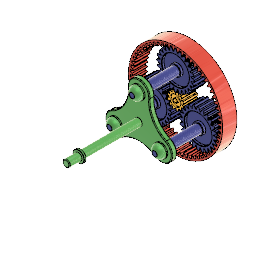
planetry gear v0 (Autodesk Fusion 360 design; units mm, degrees)
Autodesk Fusion 360 part; units mm, degrees
(part 1 of 2)
sketch "Sketch1" plane through (0, 0, 0) normal (0, 1, 0) x (1, 0, 0)
  arc A0 (-7.4766, -17.4075) -> (-18.8136, 2.2289) centre (-27.4141, -15.8275) ccw
  arc A1 (18.8136, 2.2289) -> (7.4766, -17.4075) centre (27.4141, -15.8275) ccw
  arc A2 (-11.3371, 15.1786) -> (11.3371, 15.1786) centre (0, 31.655) ccw
  arc A3 (18.8136, 2.2289) -> (11.3371, 15.1786) centre (15.5885, 9) ccw
  arc A4 (-11.3371, 15.1786) -> (-18.8136, 2.2289) centre (-15.5885, 9) ccw
  arc A5 (-7.4766, -17.4075) -> (7.4766, -17.4075) centre (0, -18) ccw
  circle A6 centre (0, -18) radius 4.5
  circle A7 centre (15.5885, 9) radius 4.5
  circle A8 centre (-15.5885, 9) radius 4.5
  circle A9 centre (0, 0) radius 2.5
  dimension "d1" = 18
  dimension "d2" = 15
  dimension "d5" = 40
  dimension "d6" = 40
  dimension "d7" = 9
  dimension "d9" = 360
  dimension "d10" = 5
  constraint tangent A1 A5
  constraint tangent A1 A3
  constraint tangent A2 A3
  constraint tangent A2 A4
  constraint concentric A5 A6
  constraint coincident A9.centre origin
  measures "d1" distance of A9.centre A5.centre
  measures "d2" diameter of A5
  measures "d5" diameter of A1
  measures "d6" diameter of A2
  measures "d7" diameter of A6
  measures "d10" diameter of A9
extrude "Extrude1" add sketch "Sketch1" along normal blind 3.5 makes body 1
extrude "Extrude2" add sketch "Sketch1" against normal blind 50 separate body contours A9 makes body 2
ref_plane "WorkPlane1" through (0, -40, 0) normal (0, 1, 0) x (0, 0, 1)
sketch "Sketch2" plane through (0, -40, 0) normal (0, 1, 0) x (1, 0, 0)
  circle A0 centre (0, 0) radius 4
  dimension "d16" = 8
  constraint coincident A0.centre origin
  measures "d16" diameter of A0
extrude "Extrude3" add sketch "Sketch2" against normal blind 1.5 bodies 2
fillet "Fillet1" radius 0.5 12 edges at (22.0836, 3.5, -12.75) (0, 3.5, -11.655) (-22.0836, 3.5, -12.75) (-10.0935, 3.5, 5.8275) (0, 3.5, 25.5) (10.0935, 3.5, 5.8275) (0, 0, 25.5) (-10.0935, 0, 5.8275) (-22.0836, 0, -12.75) (0, 0, -11.655) (22.0836, 0, -12.75) (10.0935, 0, 5.8275) on bodies 1
fillet "Fillet2" radius 0.2 2 edges at (-3.7293, -40, 1.4465) (-3.7293, -41.5, -1.4465) on bodies 2
chamfer "Chamfer1" distance 0.5 angle 45 1 edges at (-2.3308, -50, -0.904) measured on face at (-0.8863, -50, -0.2321) on bodies 2
ref_plane "WorkPlane2" through (0, 35.45, 0) normal (0, 1, 0) x (0, 0, 1)
sketch "Sketch3" plane through (0, 35.45, 0) normal (0, 1, 0) x (1, 0, 0)
  line L0 (0.5196, -30.9896) -> (0.9976, -29.763)
  arc A0 (0.9976, -29.763) -> (1.2198, -28.6806) centre (-2.0612, -28.571) ccw
  line L1 (0, -31.1) -> (0, -31.7)
  line L2 (-0.5196, -30.9896) -> (-0.9976, -29.763)
  arc A1 (-1.2198, -28.6806) -> (-0.9976, -29.763) centre (2.0612, -28.571) ccw
  arc A2 (-0.5196, -30.9896) -> (0.5196, -30.9896) centre (0, -18) ccw
  arc A3 (4.0081, -29.104) -> (3.9426, -28.0009) centre (0.745, -28.7442) ccw
  line L3 (3.8638, -30.4125) -> (4.0081, -29.104)
  arc A4 (2.8601, -30.6815) -> (3.8638, -30.4125) centre (0, -18) ccw
  line L4 (2.8601, -30.6815) -> (2.0809, -29.6204)
  arc A5 (1.5861, -28.6324) -> (2.0809, -29.6204) centre (4.7269, -27.6773) ccw
  arc A6 (6.7454, -27.6882) -> (6.3967, -26.6397) centre (3.5005, -28.1853) ccw
  line L5 (6.9448, -28.9895) -> (6.7454, -27.6882)
  arc A7 (6.0448, -29.5091) -> (6.9448, -28.9895) centre (0, -18) ccw
  line L6 (6.0448, -29.5091) -> (5.0175, -28.6858)
  arc A8 (4.2839, -27.8596) -> (5.0175, -28.6858) centre (7.0705, -26.1241) ccw
  arc A9 (9.0231, -25.6123) -> (8.4149, -24.6897) centre (6.0173, -26.9323) ccw
  line L7 (9.5524, -26.8176) -> (9.0231, -25.6123)
  arc A10 (8.8176, -27.5524) -> (9.5524, -26.8176) centre (0, -18) ccw
  line L8 (8.8176, -27.5524) -> (7.6123, -27.0231)
  arc A11 (6.6897, -26.4149) -> (7.6123, -27.0231) centre (8.9323, -24.0173) ccw
  arc A12 (10.6858, -23.0175) -> (9.8596, -22.2839) centre (8.1241, -25.0705) ccw
  line L9 (11.5091, -24.0448) -> (10.6858, -23.0175)
  arc A13 (10.9895, -24.9448) -> (11.5091, -24.0448) centre (0, -18) ccw
  line L10 (10.9895, -24.9448) -> (9.6882, -24.7454)
  arc A14 (8.6397, -24.3967) -> (9.6882, -24.7454) centre (10.1853, -21.5005) ccw
  arc A15 (11.6204, -20.0809) -> (10.6324, -19.5861) centre (9.6773, -22.7269) ccw
  line L11 (12.6815, -20.8601) -> (11.6204, -20.0809)
  arc A16 (12.4125, -21.8638) -> (12.6815, -20.8601) centre (0, -18) ccw
  line L12 (12.4125, -21.8638) -> (11.104, -22.0081)
  arc A17 (10.0009, -21.9426) -> (11.104, -22.0081) centre (10.7442, -18.745) ccw
  arc A18 (11.763, -17.0024) -> (10.6806, -16.7802) centre (10.571, -20.0612) ccw
  line L13 (12.9896, -17.4804) -> (11.763, -17.0024)
  arc A19 (12.9896, -18.5196) -> (12.9896, -17.4804) centre (0, -18) ccw
  line L14 (12.9896, -18.5196) -> (11.763, -18.9976)
  arc A20 (10.6806, -19.2198) -> (11.763, -18.9976) centre (10.571, -15.9388) ccw
  arc A21 (11.104, -13.9919) -> (10.0009, -14.0574) centre (10.7442, -17.255) ccw
  line L15 (12.4125, -14.1362) -> (11.104, -13.9919)
  arc A22 (12.6815, -15.1399) -> (12.4125, -14.1362) centre (0, -18) ccw
  line L16 (12.6815, -15.1399) -> (11.6204, -15.9191)
  arc A23 (10.6324, -16.4139) -> (11.6204, -15.9191) centre (9.6773, -13.2731) ccw
  arc A24 (9.6882, -11.2546) -> (8.6397, -11.6033) centre (10.1853, -14.4995) ccw
  line L17 (10.9895, -11.0552) -> (9.6882, -11.2546)
  arc A25 (11.5091, -11.9552) -> (10.9895, -11.0552) centre (0, -18) ccw
  line L18 (11.5091, -11.9552) -> (10.6858, -12.9825)
  arc A26 (9.8596, -13.7161) -> (10.6858, -12.9825) centre (8.1241, -10.9295) ccw
  arc A27 (7.6123, -8.9769) -> (6.6897, -9.5851) centre (8.9323, -11.9827) ccw
  line L19 (8.8176, -8.4476) -> (7.6123, -8.9769)
  arc A28 (9.5524, -9.1824) -> (8.8176, -8.4476) centre (0, -18) ccw
  line L20 (9.5524, -9.1824) -> (9.0231, -10.3877)
  arc A29 (8.4149, -11.3103) -> (9.0231, -10.3877) centre (6.0173, -9.0677) ccw
  arc A30 (5.0175, -7.3142) -> (4.2839, -8.1404) centre (7.0705, -9.8759) ccw
  line L21 (6.0448, -6.4909) -> (5.0175, -7.3142)
  arc A31 (6.9448, -7.0105) -> (6.0448, -6.4909) centre (0, -18) ccw
  line L22 (6.9448, -7.0105) -> (6.7454, -8.3118)
  arc A32 (6.3967, -9.3603) -> (6.7454, -8.3118) centre (3.5005, -7.8147) ccw
  arc A33 (2.0809, -6.3796) -> (1.5861, -7.3676) centre (4.7269, -8.3227) ccw
  line L23 (2.8601, -5.3185) -> (2.0809, -6.3796)
  arc A34 (3.8638, -5.5875) -> (2.8601, -5.3185) centre (0, -18) ccw
  line L24 (3.8638, -5.5875) -> (4.0081, -6.896)
  arc A35 (3.9426, -7.9991) -> (4.0081, -6.896) centre (0.745, -7.2558) ccw
  arc A36 (-0.9976, -6.237) -> (-1.2198, -7.3194) centre (2.0612, -7.429) ccw
  line L25 (-0.5196, -5.0104) -> (-0.9976, -6.237)
  arc A37 (0.5196, -5.0104) -> (-0.5196, -5.0104) centre (0, -18) ccw
  line L26 (0.5196, -5.0104) -> (0.9976, -6.237)
  arc A38 (1.2198, -7.3194) -> (0.9976, -6.237) centre (-2.0612, -7.429) ccw
  arc A39 (-4.0081, -6.896) -> (-3.9426, -7.9991) centre (-0.745, -7.2558) ccw
  line L27 (-3.8638, -5.5875) -> (-4.0081, -6.896)
  arc A40 (-2.8601, -5.3185) -> (-3.8638, -5.5875) centre (0, -18) ccw
  line L28 (-2.8601, -5.3185) -> (-2.0809, -6.3796)
  arc A41 (-1.5861, -7.3676) -> (-2.0809, -6.3796) centre (-4.7269, -8.3227) ccw
  arc A42 (-6.7454, -8.3118) -> (-6.3967, -9.3603) centre (-3.5005, -7.8147) ccw
  line L29 (-6.9448, -7.0105) -> (-6.7454, -8.3118)
  arc A43 (-6.0448, -6.4909) -> (-6.9448, -7.0105) centre (0, -18) ccw
  line L30 (-6.0448, -6.4909) -> (-5.0175, -7.3142)
  arc A44 (-4.2839, -8.1404) -> (-5.0175, -7.3142) centre (-7.0705, -9.8759) ccw
  arc A45 (-9.0231, -10.3877) -> (-8.4149, -11.3103) centre (-6.0173, -9.0677) ccw
  line L31 (-9.5524, -9.1824) -> (-9.0231, -10.3877)
  arc A46 (-8.8176, -8.4476) -> (-9.5524, -9.1824) centre (0, -18) ccw
  line L32 (-8.8176, -8.4476) -> (-7.6123, -8.9769)
  arc A47 (-6.6897, -9.5851) -> (-7.6123, -8.9769) centre (-8.9323, -11.9827) ccw
  arc A48 (-10.6858, -12.9825) -> (-9.8596, -13.7161) centre (-8.1241, -10.9295) ccw
  line L33 (-11.5091, -11.9552) -> (-10.6858, -12.9825)
  arc A49 (-10.9895, -11.0552) -> (-11.5091, -11.9552) centre (0, -18) ccw
  line L34 (-10.9895, -11.0552) -> (-9.6882, -11.2546)
  arc A50 (-8.6397, -11.6033) -> (-9.6882, -11.2546) centre (-10.1853, -14.4995) ccw
  arc A51 (-11.6204, -15.9191) -> (-10.6324, -16.4139) centre (-9.6773, -13.2731) ccw
  line L35 (-12.6815, -15.1399) -> (-11.6204, -15.9191)
  arc A52 (-12.4125, -14.1362) -> (-12.6815, -15.1399) centre (0, -18) ccw
  line L36 (-12.4125, -14.1362) -> (-11.104, -13.9919)
  arc A53 (-10.0009, -14.0574) -> (-11.104, -13.9919) centre (-10.7442, -17.255) ccw
  arc A54 (-11.763, -18.9976) -> (-10.6806, -19.2198) centre (-10.571, -15.9388) ccw
  line L37 (-12.9896, -18.5196) -> (-11.763, -18.9976)
  arc A55 (-12.9896, -17.4804) -> (-12.9896, -18.5196) centre (0, -18) ccw
  line L38 (-12.9896, -17.4804) -> (-11.763, -17.0024)
  arc A56 (-10.6806, -16.7802) -> (-11.763, -17.0024) centre (-10.571, -20.0612) ccw
  arc A57 (-11.104, -22.0081) -> (-10.0009, -21.9426) centre (-10.7442, -18.745) ccw
  line L39 (-12.4125, -21.8638) -> (-11.104, -22.0081)
  arc A58 (-12.6815, -20.8601) -> (-12.4125, -21.8638) centre (0, -18) ccw
  line L40 (-12.6815, -20.8601) -> (-11.6204, -20.0809)
  arc A59 (-10.6324, -19.5861) -> (-11.6204, -20.0809) centre (-9.6773, -22.7269) ccw
  arc A60 (-9.6882, -24.7454) -> (-8.6397, -24.3967) centre (-10.1853, -21.5005) ccw
  line L41 (-10.9895, -24.9448) -> (-9.6882, -24.7454)
  arc A61 (-11.5091, -24.0448) -> (-10.9895, -24.9448) centre (0, -18) ccw
  line L42 (-11.5091, -24.0448) -> (-10.6858, -23.0175)
  arc A62 (-9.8596, -22.2839) -> (-10.6858, -23.0175) centre (-8.1241, -25.0705) ccw
  arc A63 (-7.6123, -27.0231) -> (-6.6897, -26.4149) centre (-8.9323, -24.0173) ccw
  line L43 (-8.8176, -27.5524) -> (-7.6123, -27.0231)
  arc A64 (-9.5524, -26.8176) -> (-8.8176, -27.5524) centre (0, -18) ccw
  line L44 (-9.5524, -26.8176) -> (-9.0231, -25.6123)
  arc A65 (-8.4149, -24.6897) -> (-9.0231, -25.6123) centre (-6.0173, -26.9323) ccw
  arc A66 (-5.0175, -28.6858) -> (-4.2839, -27.8596) centre (-7.0705, -26.1241) ccw
  line L45 (-6.0448, -29.5091) -> (-5.0175, -28.6858)
  arc A67 (-6.9448, -28.9895) -> (-6.0448, -29.5091) centre (0, -18) ccw
  line L46 (-6.9448, -28.9895) -> (-6.7454, -27.6882)
  arc A68 (-6.3967, -26.6397) -> (-6.7454, -27.6882) centre (-3.5005, -28.1853) ccw
  arc A69 (-2.0809, -29.6204) -> (-1.5861, -28.6324) centre (-4.7269, -27.6773) ccw
  line L47 (-2.8601, -30.6815) -> (-2.0809, -29.6204)
  arc A70 (-3.8638, -30.4125) -> (-2.8601, -30.6815) centre (0, -18) ccw
  line L48 (-3.8638, -30.4125) -> (-4.0081, -29.104)
  arc A71 (-3.9426, -28.0009) -> (-4.0081, -29.104) centre (-0.745, -28.7442) ccw
  arc A72 (-1.5861, -28.6324) -> (-1.2198, -28.6806) centre (0, -18) ccw
  arc A73 (1.2198, -28.6806) -> (1.5861, -28.6324) centre (0, -18) ccw
  arc A74 (-4.2839, -27.8596) -> (-3.9426, -28.0009) centre (0, -18) ccw
  arc A75 (-6.6897, -26.4149) -> (-6.3967, -26.6397) centre (0, -18) ccw
  arc A76 (3.9426, -28.0009) -> (4.2839, -27.8596) centre (0, -18) ccw
  arc A77 (6.3967, -26.6397) -> (6.6897, -26.4149) centre (0, -18) ccw
  arc A78 (8.4149, -24.6897) -> (8.6397, -24.3967) centre (0, -18) ccw
  arc A79 (9.8596, -22.2839) -> (10.0009, -21.9426) centre (0, -18) ccw
  arc A80 (10.6324, -19.5861) -> (10.6806, -19.2198) centre (0, -18) ccw
  arc A81 (10.6806, -16.7802) -> (10.6324, -16.4139) centre (0, -18) ccw
  arc A82 (10.0009, -14.0574) -> (9.8596, -13.7161) centre (0, -18) ccw
  arc A83 (8.6397, -11.6033) -> (8.4149, -11.3103) centre (0, -18) ccw
  arc A84 (6.6897, -9.5851) -> (6.3967, -9.3603) centre (0, -18) ccw
  arc A85 (4.2839, -8.1404) -> (3.9426, -7.9991) centre (0, -18) ccw
  arc A86 (1.5861, -7.3676) -> (1.2198, -7.3194) centre (0, -18) ccw
  arc A87 (-1.2198, -7.3194) -> (-1.5861, -7.3676) centre (0, -18) ccw
  arc A88 (-3.9426, -7.9991) -> (-4.2839, -8.1404) centre (0, -18) ccw
  arc A89 (-6.3967, -9.3603) -> (-6.6897, -9.5851) centre (0, -18) ccw
  arc A90 (-8.4149, -11.3103) -> (-8.6397, -11.6033) centre (0, -18) ccw
  arc A91 (-9.8596, -13.7161) -> (-10.0009, -14.0574) centre (0, -18) ccw
  arc A92 (-10.6324, -16.4139) -> (-10.6806, -16.7802) centre (0, -18) ccw
  arc A93 (-10.6806, -19.2198) -> (-10.6324, -19.5861) centre (0, -18) ccw
  arc A94 (-10.0009, -21.9426) -> (-9.8596, -22.2839) centre (0, -18) ccw
  arc A95 (-8.6397, -24.3967) -> (-8.4149, -24.6897) centre (0, -18) ccw
  circle A96 centre (0, -18) radius 3
  dimension "d26" = 26
  dimension "d28" = 21.5
  dimension "d32" = 360
  dimension "d33" = 6
  constraint concentric A2 A72
  constraint coincident A0.end A72
  constraint tangent L0 A0
  constraint vertical L1
  constraint symmetric L0.start L1 L2.start
  constraint symmetric L0.end L1 L2.end
  constraint symmetric A0.end L1 A1.start
  constraint symmetric A0 L1 A1
  constraint concentric A72 A73
  constraint concentric A73 A76
  constraint concentric A74 A76
  constraint concentric A75 A76
  constraint concentric A76 A77
  constraint concentric A77 A78
  constraint concentric A78 A79
  constraint concentric A79 A80
  constraint concentric A80 A81
  constraint concentric A81 A82
  constraint concentric A82 A83
  constraint concentric A83 A84
  constraint concentric A84 A85
  constraint concentric A85 A86
  constraint concentric A86 A87
  constraint concentric A87 A88
  constraint concentric A88 A89
  constraint concentric A89 A90
  constraint concentric A90 A91
  constraint concentric A91 A92
  constraint concentric A92 A93
  constraint concentric A93 A94
  constraint concentric A94 A95
  constraint concentric A22 A96
  measures "d26" diameter of A2
  measures "d28" diameter of A72
  measures "d33" diameter of A96
extrude "Extrude4" add sketch "Sketch3" against normal blind 10 separate body makes body 3
sketch "Sketch4" plane through (0, 25.45, 0) normal (0, -1, 0) x (1, 0, 0)
  circle A0 centre (0, 18) radius 3
  arc A1 (-10.9895, 24.9448) -> (-11.5091, 24.0448) centre (0, 18) ccw
  line L0 (-11.5091, 24.0448) -> (-10.6858, 23.0175)
  arc A2 (-10.6858, 23.0175) -> (-9.8596, 22.2839) centre (-8.1241, 25.0705) ccw
  arc A3 (-9.8596, 22.2839) -> (-10.0009, 21.9426) centre (0, 18) ccw
  arc A4 (-10.0009, 21.9426) -> (-11.104, 22.0081) centre (-10.7442, 18.745) ccw
  line L1 (-11.104, 22.0081) -> (-12.4125, 21.8638)
  arc A5 (-12.4125, 21.8638) -> (-12.6815, 20.8601) centre (0, 18) ccw
  line L2 (-12.6815, 20.8601) -> (-11.6204, 20.0809)
  arc A6 (-11.6204, 20.0809) -> (-10.6324, 19.5861) centre (-9.6773, 22.7269) ccw
  arc A7 (-10.6324, 19.5861) -> (-10.6806, 19.2198) centre (0, 18) ccw
  arc A8 (-10.6806, 19.2198) -> (-11.763, 18.9976) centre (-10.571, 15.9388) ccw
  line L3 (-11.763, 18.9976) -> (-12.9896, 18.5196)
  arc A9 (-12.9896, 18.5196) -> (-12.9896, 17.4804) centre (0, 18) ccw
  line L4 (-12.9896, 17.4804) -> (-11.763, 17.0024)
  arc A10 (-11.763, 17.0024) -> (-10.6806, 16.7802) centre (-10.571, 20.0612) ccw
  arc A11 (-10.6806, 16.7802) -> (-10.6324, 16.4139) centre (0, 18) ccw
  arc A12 (-10.6324, 16.4139) -> (-11.6204, 15.9191) centre (-9.6773, 13.2731) ccw
  line L5 (-11.6204, 15.9191) -> (-12.6815, 15.1399)
  arc A13 (-12.6815, 15.1399) -> (-12.4125, 14.1362) centre (0, 18) ccw
  line L6 (-12.4125, 14.1362) -> (-11.104, 13.9919)
  arc A14 (-11.104, 13.9919) -> (-10.0009, 14.0574) centre (-10.7442, 17.255) ccw
  arc A15 (-10.0009, 14.0574) -> (-9.8596, 13.7161) centre (0, 18) ccw
  arc A16 (-9.8596, 13.7161) -> (-10.6858, 12.9825) centre (-8.1241, 10.9295) ccw
  line L7 (-10.6858, 12.9825) -> (-11.5091, 11.9552)
  arc A17 (-11.5091, 11.9552) -> (-10.9895, 11.0552) centre (0, 18) ccw
  line L8 (-10.9895, 11.0552) -> (-9.6882, 11.2546)
  arc A18 (-9.6882, 11.2546) -> (-8.6397, 11.6033) centre (-10.1853, 14.4995) ccw
  arc A19 (-8.6397, 11.6033) -> (-8.4149, 11.3103) centre (0, 18) ccw
  arc A20 (-8.4149, 11.3103) -> (-9.0231, 10.3877) centre (-6.0173, 9.0677) ccw
  line L9 (-9.0231, 10.3877) -> (-9.5524, 9.1824)
  arc A21 (-9.5524, 9.1824) -> (-8.8176, 8.4476) centre (0, 18) ccw
  line L10 (-8.8176, 8.4476) -> (-7.6123, 8.9769)
  arc A22 (-7.6123, 8.9769) -> (-6.6897, 9.5851) centre (-8.9323, 11.9827) ccw
  arc A23 (-6.6897, 9.5851) -> (-6.3967, 9.3603) centre (0, 18) ccw
  arc A24 (-6.3967, 9.3603) -> (-6.7454, 8.3118) centre (-3.5005, 7.8147) ccw
  line L11 (-6.7454, 8.3118) -> (-6.9448, 7.0105)
  arc A25 (-6.9448, 7.0105) -> (-6.0448, 6.4909) centre (0, 18) ccw
  line L12 (-6.0448, 6.4909) -> (-5.0175, 7.3142)
  arc A26 (-5.0175, 7.3142) -> (-4.2839, 8.1404) centre (-7.0705, 9.8759) ccw
  arc A27 (-4.2839, 8.1404) -> (-3.9426, 7.9991) centre (0, 18) ccw
  arc A28 (-3.9426, 7.9991) -> (-4.0081, 6.896) centre (-0.745, 7.2558) ccw
  line L13 (-4.0081, 6.896) -> (-3.8638, 5.5875)
  arc A29 (-3.8638, 5.5875) -> (-2.8601, 5.3185) centre (0, 18) ccw
  line L14 (-2.8601, 5.3185) -> (-2.0809, 6.3796)
  arc A30 (-2.0809, 6.3796) -> (-1.5861, 7.3676) centre (-4.7269, 8.3227) ccw
  arc A31 (-1.5861, 7.3676) -> (-1.2198, 7.3194) centre (0, 18) ccw
  arc A32 (-1.2198, 7.3194) -> (-0.9976, 6.237) centre (2.0612, 7.429) ccw
  line L15 (-0.9976, 6.237) -> (-0.5196, 5.0104)
  arc A33 (-0.5196, 5.0104) -> (0.5196, 5.0104) centre (0, 18) ccw
  line L16 (0.5196, 5.0104) -> (0.9976, 6.237)
  arc A34 (0.9976, 6.237) -> (1.2198, 7.3194) centre (-2.0612, 7.429) ccw
  arc A35 (1.2198, 7.3194) -> (1.5861, 7.3676) centre (0, 18) ccw
  arc A36 (1.5861, 7.3676) -> (2.0809, 6.3796) centre (4.7269, 8.3227) ccw
  line L17 (2.0809, 6.3796) -> (2.8601, 5.3185)
  arc A37 (2.8601, 5.3185) -> (3.8638, 5.5875) centre (0, 18) ccw
  line L18 (3.8638, 5.5875) -> (4.0081, 6.896)
  arc A38 (4.0081, 6.896) -> (3.9426, 7.9991) centre (0.745, 7.2558) ccw
  arc A39 (3.9426, 7.9991) -> (4.2839, 8.1404) centre (0, 18) ccw
  arc A40 (4.2839, 8.1404) -> (5.0175, 7.3142) centre (7.0705, 9.8759) ccw
  line L19 (5.0175, 7.3142) -> (6.0448, 6.4909)
  arc A41 (6.0448, 6.4909) -> (6.9448, 7.0105) centre (0, 18) ccw
  line L20 (6.9448, 7.0105) -> (6.7454, 8.3118)
  arc A42 (6.7454, 8.3118) -> (6.3967, 9.3603) centre (3.5005, 7.8147) ccw
  arc A43 (6.3967, 9.3603) -> (6.6897, 9.5851) centre (0, 18) ccw
  arc A44 (6.6897, 9.5851) -> (7.6123, 8.9769) centre (8.9323, 11.9827) ccw
  line L21 (7.6123, 8.9769) -> (8.8176, 8.4476)
  arc A45 (8.8176, 8.4476) -> (9.5524, 9.1824) centre (0, 18) ccw
  line L22 (9.5524, 9.1824) -> (9.0231, 10.3877)
  arc A46 (9.0231, 10.3877) -> (8.4149, 11.3103) centre (6.0173, 9.0677) ccw
  arc A47 (8.4149, 11.3103) -> (8.6397, 11.6033) centre (0, 18) ccw
  arc A48 (8.6397, 11.6033) -> (9.6882, 11.2546) centre (10.1853, 14.4995) ccw
  line L23 (9.6882, 11.2546) -> (10.9895, 11.0552)
  arc A49 (10.9895, 11.0552) -> (11.5091, 11.9552) centre (0, 18) ccw
  line L24 (11.5091, 11.9552) -> (10.6858, 12.9825)
  arc A50 (10.6858, 12.9825) -> (9.8596, 13.7161) centre (8.1241, 10.9295) ccw
  arc A51 (9.8596, 13.7161) -> (10.0009, 14.0574) centre (0, 18) ccw
  arc A52 (10.0009, 14.0574) -> (11.104, 13.9919) centre (10.7442, 17.255) ccw
  line L25 (11.104, 13.9919) -> (12.4125, 14.1362)
  arc A53 (12.4125, 14.1362) -> (12.6815, 15.1399) centre (0, 18) ccw
  line L26 (12.6815, 15.1399) -> (11.6204, 15.9191)
  arc A54 (11.6204, 15.9191) -> (10.6324, 16.4139) centre (9.6773, 13.2731) ccw
  arc A55 (10.6324, 16.4139) -> (10.6806, 16.7802) centre (0, 18) ccw
  arc A56 (10.6806, 16.7802) -> (11.763, 17.0024) centre (10.571, 20.0612) ccw
  line L27 (11.763, 17.0024) -> (12.9896, 17.4804)
  arc A57 (12.9896, 17.4804) -> (12.9896, 18.5196) centre (0, 18) ccw
  line L28 (12.9896, 18.5196) -> (11.763, 18.9976)
  arc A58 (11.763, 18.9976) -> (10.6806, 19.2198) centre (10.571, 15.9388) ccw
  arc A59 (10.6806, 19.2198) -> (10.6324, 19.5861) centre (0, 18) ccw
  arc A60 (10.6324, 19.5861) -> (11.6204, 20.0809) centre (9.6773, 22.7269) ccw
  line L29 (11.6204, 20.0809) -> (12.6815, 20.8601)
  arc A61 (12.6815, 20.8601) -> (12.4125, 21.8638) centre (0, 18) ccw
  line L30 (12.4125, 21.8638) -> (11.104, 22.0081)
  arc A62 (11.104, 22.0081) -> (10.0009, 21.9426) centre (10.7442, 18.745) ccw
  arc A63 (10.0009, 21.9426) -> (9.8596, 22.2839) centre (0, 18) ccw
  arc A64 (9.8596, 22.2839) -> (10.6858, 23.0175) centre (8.1241, 25.0705) ccw
  line L31 (10.6858, 23.0175) -> (11.5091, 24.0448)
  arc A65 (11.5091, 24.0448) -> (10.9895, 24.9448) centre (0, 18) ccw
  line L32 (10.9895, 24.9448) -> (9.6882, 24.7454)
  arc A66 (9.6882, 24.7454) -> (8.6397, 24.3967) centre (10.1853, 21.5005) ccw
  arc A67 (8.6397, 24.3967) -> (8.4149, 24.6897) centre (0, 18) ccw
  arc A68 (8.4149, 24.6897) -> (9.0231, 25.6123) centre (6.0173, 26.9323) ccw
  line L33 (9.0231, 25.6123) -> (9.5524, 26.8176)
  arc A69 (9.5524, 26.8176) -> (8.8176, 27.5524) centre (0, 18) ccw
  line L34 (8.8176, 27.5524) -> (7.6123, 27.0231)
  arc A70 (7.6123, 27.0231) -> (6.6897, 26.4149) centre (8.9323, 24.0173) ccw
  arc A71 (6.6897, 26.4149) -> (6.3967, 26.6397) centre (0, 18) ccw
  arc A72 (6.3967, 26.6397) -> (6.7454, 27.6882) centre (3.5005, 28.1853) ccw
  line L35 (6.7454, 27.6882) -> (6.9448, 28.9895)
  arc A73 (6.9448, 28.9895) -> (6.0448, 29.5091) centre (0, 18) ccw
  line L36 (6.0448, 29.5091) -> (5.0175, 28.6858)
  arc A74 (5.0175, 28.6858) -> (4.2839, 27.8596) centre (7.0705, 26.1241) ccw
  arc A75 (4.2839, 27.8596) -> (3.9426, 28.0009) centre (0, 18) ccw
  arc A76 (3.9426, 28.0009) -> (4.0081, 29.104) centre (0.745, 28.7442) ccw
  line L37 (4.0081, 29.104) -> (3.8638, 30.4125)
  arc A77 (3.8638, 30.4125) -> (2.8601, 30.6815) centre (0, 18) ccw
  line L38 (2.8601, 30.6815) -> (2.0809, 29.6204)
  arc A78 (2.0809, 29.6204) -> (1.5861, 28.6324) centre (4.7269, 27.6773) ccw
  arc A79 (1.5861, 28.6324) -> (1.2198, 28.6806) centre (0, 18) ccw
  arc A80 (1.2198, 28.6806) -> (0.9976, 29.763) centre (-2.0612, 28.571) ccw
  line L39 (0.9976, 29.763) -> (0.5196, 30.9896)
  arc A81 (0.5196, 30.9896) -> (-0.5196, 30.9896) centre (0, 18) ccw
  line L40 (-0.5196, 30.9896) -> (-0.9976, 29.763)
  arc A82 (-0.9976, 29.763) -> (-1.2198, 28.6806) centre (2.0612, 28.571) ccw
  arc A83 (-1.2198, 28.6806) -> (-1.5861, 28.6324) centre (0, 18) ccw
  arc A84 (-1.5861, 28.6324) -> (-2.0809, 29.6204) centre (-4.7269, 27.6773) ccw
  line L41 (-2.0809, 29.6204) -> (-2.8601, 30.6815)
  arc A85 (-2.8601, 30.6815) -> (-3.8638, 30.4125) centre (0, 18) ccw
  line L42 (-3.8638, 30.4125) -> (-4.0081, 29.104)
  arc A86 (-4.0081, 29.104) -> (-3.9426, 28.0009) centre (-0.745, 28.7442) ccw
  arc A87 (-3.9426, 28.0009) -> (-4.2839, 27.8596) centre (0, 18) ccw
  arc A88 (-4.2839, 27.8596) -> (-5.0175, 28.6858) centre (-7.0705, 26.1241) ccw
  line L43 (-5.0175, 28.6858) -> (-6.0448, 29.5091)
  arc A89 (-6.0448, 29.5091) -> (-6.9448, 28.9895) centre (0, 18) ccw
  line L44 (-6.9448, 28.9895) -> (-6.7454, 27.6882)
  arc A90 (-6.7454, 27.6882) -> (-6.3967, 26.6397) centre (-3.5005, 28.1853) ccw
  arc A91 (-6.3967, 26.6397) -> (-6.6897, 26.4149) centre (0, 18) ccw
  arc A92 (-6.6897, 26.4149) -> (-7.6123, 27.0231) centre (-8.9323, 24.0173) ccw
  line L45 (-7.6123, 27.0231) -> (-8.8176, 27.5524)
  arc A93 (-8.8176, 27.5524) -> (-9.5524, 26.8176) centre (0, 18) ccw
  line L46 (-9.5524, 26.8176) -> (-9.0231, 25.6123)
  arc A94 (-9.0231, 25.6123) -> (-8.4149, 24.6897) centre (-6.0173, 26.9323) ccw
  arc A95 (-8.4149, 24.6897) -> (-8.6397, 24.3967) centre (0, 18) ccw
  arc A96 (-8.6397, 24.3967) -> (-9.6882, 24.7454) centre (-10.1853, 21.5005) ccw
  line L47 (-9.6882, 24.7454) -> (-10.9895, 24.9448)
  circle A97 centre (0, 18) radius 9.375
  circle A98 centre (0, 18) radius 3.75
  dimension "d36" = 18.75
  dimension "d37" = 7.5
  constraint concentric A0 A97
  constraint concentric A97 A98
  measures "d36" diameter of A97
  measures "d37" diameter of A98
extrude "Extrude5" cut sketch "Sketch4" against normal blind 1.5 contours A97 bodies 3
sketch "Sketch5" plane through (0, 35.45, 0) normal (0, 1, 0) x (-1, 0, 0)
  circle A0 centre (0, 18) radius 3
  arc A1 (11.5091, 24.0448) -> (10.9895, 24.9448) centre (0, 18) ccw
  line L0 (10.9895, 24.9448) -> (9.6882, 24.7454)
  arc A2 (9.6882, 24.7454) -> (8.6397, 24.3967) centre (10.1853, 21.5005) ccw
  arc A3 (8.6397, 24.3967) -> (8.4149, 24.6897) centre (0, 18) ccw
  arc A4 (8.4149, 24.6897) -> (9.0231, 25.6123) centre (6.0173, 26.9323) ccw
  line L1 (9.0231, 25.6123) -> (9.5524, 26.8176)
  arc A5 (9.5524, 26.8176) -> (8.8176, 27.5524) centre (0, 18) ccw
  line L2 (8.8176, 27.5524) -> (7.6123, 27.0231)
  arc A6 (7.6123, 27.0231) -> (6.6897, 26.4149) centre (8.9323, 24.0173) ccw
  arc A7 (6.6897, 26.4149) -> (6.3967, 26.6397) centre (0, 18) ccw
  arc A8 (6.3967, 26.6397) -> (6.7454, 27.6882) centre (3.5005, 28.1853) ccw
  line L3 (6.7454, 27.6882) -> (6.9448, 28.9895)
  arc A9 (6.9448, 28.9895) -> (6.0448, 29.5091) centre (0, 18) ccw
  line L4 (6.0448, 29.5091) -> (5.0175, 28.6858)
  arc A10 (5.0175, 28.6858) -> (4.2839, 27.8596) centre (7.0705, 26.1241) ccw
  arc A11 (4.2839, 27.8596) -> (3.9426, 28.0009) centre (0, 18) ccw
  arc A12 (3.9426, 28.0009) -> (4.0081, 29.104) centre (0.745, 28.7442) ccw
  line L5 (4.0081, 29.104) -> (3.8638, 30.4125)
  arc A13 (3.8638, 30.4125) -> (2.8601, 30.6815) centre (0, 18) ccw
  line L6 (2.8601, 30.6815) -> (2.0809, 29.6204)
  arc A14 (2.0809, 29.6204) -> (1.5861, 28.6324) centre (4.7269, 27.6773) ccw
  arc A15 (1.5861, 28.6324) -> (1.2198, 28.6806) centre (0, 18) ccw
  arc A16 (1.2198, 28.6806) -> (0.9976, 29.763) centre (-2.0612, 28.571) ccw
  line L7 (0.9976, 29.763) -> (0.5196, 30.9896)
  arc A17 (0.5196, 30.9896) -> (-0.5196, 30.9896) centre (0, 18) ccw
  line L8 (-0.5196, 30.9896) -> (-0.9976, 29.763)
  arc A18 (-0.9976, 29.763) -> (-1.2198, 28.6806) centre (2.0612, 28.571) ccw
  arc A19 (-1.2198, 28.6806) -> (-1.5861, 28.6324) centre (0, 18) ccw
  arc A20 (-1.5861, 28.6324) -> (-2.0809, 29.6204) centre (-4.7269, 27.6773) ccw
  line L9 (-2.0809, 29.6204) -> (-2.8601, 30.6815)
  arc A21 (-2.8601, 30.6815) -> (-3.8638, 30.4125) centre (0, 18) ccw
  line L10 (-3.8638, 30.4125) -> (-4.0081, 29.104)
  arc A22 (-4.0081, 29.104) -> (-3.9426, 28.0009) centre (-0.745, 28.7442) ccw
  arc A23 (-3.9426, 28.0009) -> (-4.2839, 27.8596) centre (0, 18) ccw
  arc A24 (-4.2839, 27.8596) -> (-5.0175, 28.6858) centre (-7.0705, 26.1241) ccw
  line L11 (-5.0175, 28.6858) -> (-6.0448, 29.5091)
  arc A25 (-6.0448, 29.5091) -> (-6.9448, 28.9895) centre (0, 18) ccw
  line L12 (-6.9448, 28.9895) -> (-6.7454, 27.6882)
  arc A26 (-6.7454, 27.6882) -> (-6.3967, 26.6397) centre (-3.5005, 28.1853) ccw
  arc A27 (-6.3967, 26.6397) -> (-6.6897, 26.4149) centre (0, 18) ccw
  arc A28 (-6.6897, 26.4149) -> (-7.6123, 27.0231) centre (-8.9323, 24.0173) ccw
  line L13 (-7.6123, 27.0231) -> (-8.8176, 27.5524)
  arc A29 (-8.8176, 27.5524) -> (-9.5524, 26.8176) centre (0, 18) ccw
  line L14 (-9.5524, 26.8176) -> (-9.0231, 25.6123)
  arc A30 (-9.0231, 25.6123) -> (-8.4149, 24.6897) centre (-6.0173, 26.9323) ccw
  arc A31 (-8.4149, 24.6897) -> (-8.6397, 24.3967) centre (0, 18) ccw
  arc A32 (-8.6397, 24.3967) -> (-9.6882, 24.7454) centre (-10.1853, 21.5005) ccw
  line L15 (-9.6882, 24.7454) -> (-10.9895, 24.9448)
  arc A33 (-10.9895, 24.9448) -> (-11.5091, 24.0448) centre (0, 18) ccw
  line L16 (-11.5091, 24.0448) -> (-10.6858, 23.0175)
  arc A34 (-10.6858, 23.0175) -> (-9.8596, 22.2839) centre (-8.1241, 25.0705) ccw
  arc A35 (-9.8596, 22.2839) -> (-10.0009, 21.9426) centre (0, 18) ccw
  arc A36 (-10.0009, 21.9426) -> (-11.104, 22.0081) centre (-10.7442, 18.745) ccw
  line L17 (-11.104, 22.0081) -> (-12.4125, 21.8638)
  arc A37 (-12.4125, 21.8638) -> (-12.6815, 20.8601) centre (0, 18) ccw
  line L18 (-12.6815, 20.8601) -> (-11.6204, 20.0809)
  arc A38 (-11.6204, 20.0809) -> (-10.6324, 19.5861) centre (-9.6773, 22.7269) ccw
  arc A39 (-10.6324, 19.5861) -> (-10.6806, 19.2198) centre (0, 18) ccw
  arc A40 (-10.6806, 19.2198) -> (-11.763, 18.9976) centre (-10.571, 15.9388) ccw
  line L19 (-11.763, 18.9976) -> (-12.9896, 18.5196)
  arc A41 (-12.9896, 18.5196) -> (-12.9896, 17.4804) centre (0, 18) ccw
  line L20 (-12.9896, 17.4804) -> (-11.763, 17.0024)
  arc A42 (-11.763, 17.0024) -> (-10.6806, 16.7802) centre (-10.571, 20.0612) ccw
  arc A43 (-10.6806, 16.7802) -> (-10.6324, 16.4139) centre (0, 18) ccw
  arc A44 (-10.6324, 16.4139) -> (-11.6204, 15.9191) centre (-9.6773, 13.2731) ccw
  line L21 (-11.6204, 15.9191) -> (-12.6815, 15.1399)
  arc A45 (-12.6815, 15.1399) -> (-12.4125, 14.1362) centre (0, 18) ccw
  line L22 (-12.4125, 14.1362) -> (-11.104, 13.9919)
  arc A46 (-11.104, 13.9919) -> (-10.0009, 14.0574) centre (-10.7442, 17.255) ccw
  arc A47 (-10.0009, 14.0574) -> (-9.8596, 13.7161) centre (0, 18) ccw
  arc A48 (-9.8596, 13.7161) -> (-10.6858, 12.9825) centre (-8.1241, 10.9295) ccw
  line L23 (-10.6858, 12.9825) -> (-11.5091, 11.9552)
  arc A49 (-11.5091, 11.9552) -> (-10.9895, 11.0552) centre (0, 18) ccw
  line L24 (-10.9895, 11.0552) -> (-9.6882, 11.2546)
  arc A50 (-9.6882, 11.2546) -> (-8.6397, 11.6033) centre (-10.1853, 14.4995) ccw
  arc A51 (-8.6397, 11.6033) -> (-8.4149, 11.3103) centre (0, 18) ccw
  arc A52 (-8.4149, 11.3103) -> (-9.0231, 10.3877) centre (-6.0173, 9.0677) ccw
  line L25 (-9.0231, 10.3877) -> (-9.5524, 9.1824)
  arc A53 (-9.5524, 9.1824) -> (-8.8176, 8.4476) centre (0, 18) ccw
  line L26 (-8.8176, 8.4476) -> (-7.6123, 8.9769)
  arc A54 (-7.6123, 8.9769) -> (-6.6897, 9.5851) centre (-8.9323, 11.9827) ccw
  arc A55 (-6.6897, 9.5851) -> (-6.3967, 9.3603) centre (0, 18) ccw
  arc A56 (-6.3967, 9.3603) -> (-6.7454, 8.3118) centre (-3.5005, 7.8147) ccw
  line L27 (-6.7454, 8.3118) -> (-6.9448, 7.0105)
  arc A57 (-6.9448, 7.0105) -> (-6.0448, 6.4909) centre (0, 18) ccw
  line L28 (-6.0448, 6.4909) -> (-5.0175, 7.3142)
  arc A58 (-5.0175, 7.3142) -> (-4.2839, 8.1404) centre (-7.0705, 9.8759) ccw
  arc A59 (-4.2839, 8.1404) -> (-3.9426, 7.9991) centre (0, 18) ccw
  arc A60 (-3.9426, 7.9991) -> (-4.0081, 6.896) centre (-0.745, 7.2558) ccw
  line L29 (-4.0081, 6.896) -> (-3.8638, 5.5875)
  arc A61 (-3.8638, 5.5875) -> (-2.8601, 5.3185) centre (0, 18) ccw
  line L30 (-2.8601, 5.3185) -> (-2.0809, 6.3796)
  arc A62 (-2.0809, 6.3796) -> (-1.5861, 7.3676) centre (-4.7269, 8.3227) ccw
  arc A63 (-1.5861, 7.3676) -> (-1.2198, 7.3194) centre (0, 18) ccw
  arc A64 (-1.2198, 7.3194) -> (-0.9976, 6.237) centre (2.0612, 7.429) ccw
  line L31 (-0.9976, 6.237) -> (-0.5196, 5.0104)
  arc A65 (-0.5196, 5.0104) -> (0.5196, 5.0104) centre (0, 18) ccw
  line L32 (0.5196, 5.0104) -> (0.9976, 6.237)
  arc A66 (0.9976, 6.237) -> (1.2198, 7.3194) centre (-2.0612, 7.429) ccw
  arc A67 (1.2198, 7.3194) -> (1.5861, 7.3676) centre (0, 18) ccw
  arc A68 (1.5861, 7.3676) -> (2.0809, 6.3796) centre (4.7269, 8.3227) ccw
  line L33 (2.0809, 6.3796) -> (2.8601, 5.3185)
  arc A69 (2.8601, 5.3185) -> (3.8638, 5.5875) centre (0, 18) ccw
  line L34 (3.8638, 5.5875) -> (4.0081, 6.896)
  arc A70 (4.0081, 6.896) -> (3.9426, 7.9991) centre (0.745, 7.2558) ccw
  arc A71 (3.9426, 7.9991) -> (4.2839, 8.1404) centre (0, 18) ccw
  arc A72 (4.2839, 8.1404) -> (5.0175, 7.3142) centre (7.0705, 9.8759) ccw
  line L35 (5.0175, 7.3142) -> (6.0448, 6.4909)
  arc A73 (6.0448, 6.4909) -> (6.9448, 7.0105) centre (0, 18) ccw
  line L36 (6.9448, 7.0105) -> (6.7454, 8.3118)
  arc A74 (6.7454, 8.3118) -> (6.3967, 9.3603) centre (3.5005, 7.8147) ccw
  arc A75 (6.3967, 9.3603) -> (6.6897, 9.5851) centre (0, 18) ccw
  arc A76 (6.6897, 9.5851) -> (7.6123, 8.9769) centre (8.9323, 11.9827) ccw
  line L37 (7.6123, 8.9769) -> (8.8176, 8.4476)
  arc A77 (8.8176, 8.4476) -> (9.5524, 9.1824) centre (0, 18) ccw
  line L38 (9.5524, 9.1824) -> (9.0231, 10.3877)
  arc A78 (9.0231, 10.3877) -> (8.4149, 11.3103) centre (6.0173, 9.0677) ccw
  arc A79 (8.4149, 11.3103) -> (8.6397, 11.6033) centre (0, 18) ccw
  arc A80 (8.6397, 11.6033) -> (9.6882, 11.2546) centre (10.1853, 14.4995) ccw
  line L39 (9.6882, 11.2546) -> (10.9895, 11.0552)
  arc A81 (10.9895, 11.0552) -> (11.5091, 11.9552) centre (0, 18) ccw
  line L40 (11.5091, 11.9552) -> (10.6858, 12.9825)
  arc A82 (10.6858, 12.9825) -> (9.8596, 13.7161) centre (8.1241, 10.9295) ccw
  arc A83 (9.8596, 13.7161) -> (10.0009, 14.0574) centre (0, 18) ccw
  arc A84 (10.0009, 14.0574) -> (11.104, 13.9919) centre (10.7442, 17.255) ccw
  line L41 (11.104, 13.9919) -> (12.4125, 14.1362)
  arc A85 (12.4125, 14.1362) -> (12.6815, 15.1399) centre (0, 18) ccw
  line L42 (12.6815, 15.1399) -> (11.6204, 15.9191)
  arc A86 (11.6204, 15.9191) -> (10.6324, 16.4139) centre (9.6773, 13.2731) ccw
  arc A87 (10.6324, 16.4139) -> (10.6806, 16.7802) centre (0, 18) ccw
  arc A88 (10.6806, 16.7802) -> (11.763, 17.0024) centre (10.571, 20.0612) ccw
  line L43 (11.763, 17.0024) -> (12.9896, 17.4804)
  arc A89 (12.9896, 17.4804) -> (12.9896, 18.5196) centre (0, 18) ccw
  line L44 (12.9896, 18.5196) -> (11.763, 18.9976)
  arc A90 (11.763, 18.9976) -> (10.6806, 19.2198) centre (10.571, 15.9388) ccw
  arc A91 (10.6806, 19.2198) -> (10.6324, 19.5861) centre (0, 18) ccw
  arc A92 (10.6324, 19.5861) -> (11.6204, 20.0809) centre (9.6773, 22.7269) ccw
  line L45 (11.6204, 20.0809) -> (12.6815, 20.8601)
  arc A93 (12.6815, 20.8601) -> (12.4125, 21.8638) centre (0, 18) ccw
  line L46 (12.4125, 21.8638) -> (11.104, 22.0081)
  arc A94 (11.104, 22.0081) -> (10.0009, 21.9426) centre (10.7442, 18.745) ccw
  arc A95 (10.0009, 21.9426) -> (9.8596, 22.2839) centre (0, 18) ccw
  arc A96 (9.8596, 22.2839) -> (10.6858, 23.0175) centre (8.1241, 25.0705) ccw
  line L47 (10.6858, 23.0175) -> (11.5091, 24.0448)
  circle A97 centre (0, 18) radius 9.375
  circle A98 centre (0, 18) radius 3.75
extrude "Extrude6" cut sketch "Sketch5" against normal blind 1.5 contours A97 bodies 3
combine "Combine1" operation add target body 1 tool bodies 2
pattern_circular "C-Pattern1" count 3 over 360 about axis through (0, 1.75, 0) along (0, 1, 0) of bodies 3 makes body 4 at (11.4526, 26.95, -15.2321) makes body 5 at (-18.9176, 26.95, -2.3022)
sketch "Sketch6" plane through (0, 26.95, 0) normal (0, -1, 0) x (1, 0, 0)
  circle A0 centre (0, 18) radius 3.75
  circle A1 centre (0, 18) radius 9.375
  circle A2 centre (0, 18) radius 2.95
  dimension "d44" = 5.9
  constraint concentric A0 A2
  measures "d44" diameter of A2
extrude "Extrude7" add sketch "Sketch6" along normal blind 24 separate body contours A2 makes body 6
sketch "Sketch7" plane through (0, 2.95, 0) normal (0, -1, 0) x (1, 0, 0)
  circle A0 centre (0, 18) radius 2.95
  circle A1 centre (0, 18) radius 2.75
  dimension "d47" = 5.5
  constraint concentric A0 A1
  measures "d47" diameter of A1
extrude "Extrude8" add sketch "Sketch7" along normal blind 2.95 contours A1 bodies 6
sketch "Sketch8" plane through (0, 0, 0) normal (0, -1, 0) x (1, 0, 0)
  circle A0 centre (0, 18) radius 2.75
  circle A1 centre (0, 18) radius 2.07
  dimension "d50" = 4.14
  constraint concentric A0 A1
  measures "d50" diameter of A1
extrude "Extrude9" add sketch "Sketch8" along normal blind 4.55 contours A1 bodies 6
thread "Thread1" "ISO Metric profile 3.5 M3.5x0.6 M3.5x0.6 6g" major diameter 3.4165 minor diameter 2.732 pitch 0.6 angle 60 resizes the face on face at (2.0597, -1.5167, 17.7939) on bodies 6
chamfer "Chamfer2" distance 0.1 angle 45 1 edges at (-2.5639, 0, 17.0056) on bodies 6
chamfer "Chamfer3" distance 0.25 angle 45 1 edges at (-8.7406, 25.45, 21.3901) on bodies 3
chamfer "Chamfer4" distance 0.25 angle 45 2 edges at (22.8947, 25.45, -3.1255) (-14.1541, 25.45, -18.2646) on bodies 4 5
pattern_circular "C-Pattern2" count 3 over 360 about axis through (0, 0, 0) along (0, -1, 0) of bodies 6 makes body 7 at (-17.189, 18.95, -6.5219) makes body 8 at (14.2426, 18.95, -11.6251)
sketch "Sketch9" plane through (0, 0, 0) normal (0, -1, 0) x (1, 0, 0)
  circle A0 centre (0, 18) radius 4.5
  circle A1 centre (15.5885, -9) radius 4.5
  circle A2 centre (-15.5885, -9) radius 4.5
  circle A3 centre (0, 0) radius 2.5
  arc A4 (6.9781, 17.447) -> (-6.9781, 17.447) centre (0, 18) ccw
  arc A5 (-18.5986, -2.6803) -> (-6.9781, 17.447) centre (-27.4141, 15.8275) ccw
  arc A6 (-18.5986, -2.6803) -> (-11.6205, -14.7667) centre (-15.5885, -9) ccw
  arc A7 (11.6205, -14.7667) -> (-11.6205, -14.7667) centre (0, -31.655) ccw
  arc A8 (11.6205, -14.7667) -> (18.5986, -2.6803) centre (15.5885, -9) ccw
  arc A9 (6.9781, 17.447) -> (18.5986, -2.6803) centre (27.4141, 15.8275) ccw
  circle A10 centre (0, 18) radius 4.5
  circle A11 centre (0, 18) radius 1.85
  dimension "d60" = 3.7
  constraint concentric A0 A10
  constraint concentric A10 A11
  measures "d60" diameter of A11
extrude "Extrude10" add sketch "Sketch9" along normal blind 4.6 separate body contours A0 A10 makes body 9
fillet "Fillet3" radius 4 1 edges at (-4.1955, -4.6, 16.3727) on bodies 9
pattern_circular "C-Pattern3" count 3 over 360 about axis through (0, 0, 0) along (0, -1, 0) of bodies 9 makes body 10 at (-13.3714, -1.5575, -12.8401) makes body 11 at (17.8055, -1.5575, -5.1599)
sketch "Sketch10" plane through (0, 35.45, 0) normal (0, 1, 0) x (1, 0, 0)
  line L0 (0.955, -5.5867) -> (0.8578, -5.5034)
  arc A0 (0.4382, -4.7297) -> (0.8578, -5.5034) centre (1.6611, -4.5671) ccw
  arc A1 (2.0629, -4.9414) -> (1.9832, -4.3162) centre (0.7961, -4.7853) ccw
  line L1 (2.0192, -5.2959) -> (2.0629, -4.9414)
  arc A2 (0.955, -5.5867) -> (2.0192, -5.2959) centre (0, 0) ccw
  arc A3 (4.2572, -3.2479) -> (3.8756, -2.7463) centre (3.082, -3.7461) ccw
  line L2 (4.3966, -3.5768) -> (4.2572, -3.2479)
  arc A4 (3.6204, -4.3608) -> (4.3966, -3.5768) centre (0, 0) ccw
  arc A5 (2.7443, -3.877) -> (3.4946, -4.3372) centre (3.722, -3.1247) ccw
  line L3 (3.6204, -4.3608) -> (3.4946, -4.3372)
  arc A6 (5.3109, -0.6842) -> (4.7295, -0.4406) centre (4.5422, -1.7032) ccw
  line L4 (5.596, -0.8992) -> (5.3109, -0.6842)
  arc A7 (5.3157, -1.9663) -> (5.596, -0.8992) centre (0, 0) ccw
  arc A8 (4.3152, -1.9854) -> (5.195, -2.0088) centre (4.7857, -0.845) ccw
  line L5 (5.3157, -1.9663) -> (5.195, -2.0088)
  arc A9 (4.9414, 2.0629) -> (4.3162, 1.9832) centre (4.7853, 0.7961) ccw
  line L6 (5.2959, 2.0192) -> (4.9414, 2.0629)
  arc A10 (5.5867, 0.955) -> (5.2959, 2.0192) centre (0, 0) ccw
  arc A11 (4.7297, 0.4382) -> (5.5034, 0.8578) centre (4.5671, 1.6611) ccw
  line L7 (5.5867, 0.955) -> (5.5034, 0.8578)
  arc A12 (3.2479, 4.2572) -> (2.7463, 3.8756) centre (3.7461, 3.082) ccw
  line L8 (3.5768, 4.3966) -> (3.2479, 4.2572)
  arc A13 (4.3608, 3.6204) -> (3.5768, 4.3966) centre (0, 0) ccw
  arc A14 (3.877, 2.7443) -> (4.3372, 3.4946) centre (3.1247, 3.722) ccw
  line L9 (4.3608, 3.6204) -> (4.3372, 3.4946)
  arc A15 (0.6842, 5.3109) -> (0.4406, 4.7295) centre (1.7032, 4.5422) ccw
  line L10 (0.8992, 5.596) -> (0.6842, 5.3109)
  arc A16 (1.9663, 5.3157) -> (0.8992, 5.596) centre (0, 0) ccw
  arc A17 (1.9854, 4.3152) -> (2.0088, 5.195) centre (0.845, 4.7857) ccw
  line L11 (1.9663, 5.3157) -> (2.0088, 5.195)
  arc A18 (-2.0629, 4.9414) -> (-1.9832, 4.3162) centre (-0.7961, 4.7853) ccw
  line L12 (-2.0192, 5.2959) -> (-2.0629, 4.9414)
  arc A19 (-0.955, 5.5867) -> (-2.0192, 5.2959) centre (0, 0) ccw
  arc A20 (-0.4382, 4.7297) -> (-0.8578, 5.5034) centre (-1.6611, 4.5671) ccw
  line L13 (-0.955, 5.5867) -> (-0.8578, 5.5034)
  arc A21 (-4.2572, 3.2479) -> (-3.8756, 2.7463) centre (-3.082, 3.7461) ccw
  line L14 (-4.3966, 3.5768) -> (-4.2572, 3.2479)
  arc A22 (-3.6204, 4.3608) -> (-4.3966, 3.5768) centre (0, 0) ccw
  arc A23 (-2.7443, 3.877) -> (-3.4946, 4.3372) centre (-3.722, 3.1247) ccw
  line L15 (-3.6204, 4.3608) -> (-3.4946, 4.3372)
  arc A24 (-5.3109, 0.6842) -> (-4.7295, 0.4406) centre (-4.5422, 1.7032) ccw
  line L16 (-5.596, 0.8992) -> (-5.3109, 0.6842)
  arc A25 (-5.3157, 1.9663) -> (-5.596, 0.8992) centre (0, 0) ccw
  arc A26 (-4.3152, 1.9854) -> (-5.195, 2.0088) centre (-4.7857, 0.845) ccw
  line L17 (-5.3157, 1.9663) -> (-5.195, 2.0088)
  arc A27 (-4.9414, -2.0629) -> (-4.3162, -1.9832) centre (-4.7853, -0.7961) ccw
  line L18 (-5.2959, -2.0192) -> (-4.9414, -2.0629)
  arc A28 (-5.5867, -0.955) -> (-5.2959, -2.0192) centre (0, 0) ccw
  arc A29 (-4.7297, -0.4382) -> (-5.5034, -0.8578) centre (-4.5671, -1.6611) ccw
  line L19 (-5.5867, -0.955) -> (-5.5034, -0.8578)
  arc A30 (-3.2479, -4.2572) -> (-2.7463, -3.8756) centre (-3.7461, -3.082) ccw
  line L20 (-3.5768, -4.3966) -> (-3.2479, -4.2572)
  arc A31 (-4.3608, -3.6204) -> (-3.5768, -4.3966) centre (0, 0) ccw
  arc A32 (-3.877, -2.7443) -> (-4.3372, -3.4946) centre (-3.1247, -3.722) ccw
  line L21 (-4.3608, -3.6204) -> (-4.3372, -3.4946)
  arc A33 (-0.6842, -5.3109) -> (-0.4406, -4.7295) centre (-1.7032, -4.5422) ccw
  line L22 (-0.8992, -5.596) -> (-0.6842, -5.3109)
  arc A34 (-1.9663, -5.3157) -> (-0.8992, -5.596) centre (0, 0) ccw
  arc A35 (-1.9854, -4.3152) -> (-2.0088, -5.195) centre (-0.845, -4.7857) ccw
  line L23 (-1.9663, -5.3157) -> (-2.0088, -5.195)
  arc A36 (1.9832, -4.3162) -> (2.7443, -3.877) centre (0, 0) ccw
  arc A37 (-0.4406, -4.7295) -> (0.4382, -4.7297) centre (0, 0) ccw
  arc A38 (-2.7463, -3.8756) -> (-1.9854, -4.3152) centre (0, 0) ccw
  arc A39 (-4.3162, -1.9832) -> (-3.877, -2.7443) centre (0, 0) ccw
  arc A40 (-4.7295, 0.4406) -> (-4.7297, -0.4382) centre (0, 0) ccw
  arc A41 (-3.8756, 2.7463) -> (-4.3152, 1.9854) centre (0, 0) ccw
  arc A42 (-1.9832, 4.3162) -> (-2.7443, 3.877) centre (0, 0) ccw
  arc A43 (0.4406, 4.7295) -> (-0.4382, 4.7297) centre (0, 0) ccw
  arc A44 (2.7463, 3.8756) -> (1.9854, 4.3152) centre (0, 0) ccw
  arc A45 (4.3162, 1.9832) -> (3.877, 2.7443) centre (0, 0) ccw
  arc A46 (3.8756, -2.7463) -> (4.3152, -1.9854) centre (0, 0) ccw
  arc A47 (4.7295, -0.4406) -> (4.7297, 0.4382) centre (0, 0) ccw
  circle A48 centre (0, 0) radius 1.25
  dimension "d69" = 9.5
  dimension "d71" = 360
  dimension "d73" = 2.5
  constraint coincident A2.centre A4.centre
  constraint tangent L0 A0
  constraint coincident A1.end A46
  constraint concentric A36 A46
  constraint concentric A37 A46
  constraint concentric A38 A46
  constraint concentric A39 A46
  constraint concentric A40 A46
  constraint concentric A41 A46
  constraint concentric A42 A46
  constraint concentric A43 A46
  constraint concentric A44 A46
  constraint concentric A45 A46
  constraint concentric A46 A47
  constraint concentric A22 A48
  measures "d69" diameter of A46
  measures "d73" diameter of A48
extrude "Extrude11" add sketch "Sketch10" against normal blind 10 separate body makes body 12
sketch "Sketch11" plane through (0, 35.45, 0) normal (0, 1, 0) x (-1, 0, 0)
  circle A0 centre (0, 0) radius 1.25
  arc A1 (-5.3157, 1.9663) -> (-5.596, 0.8992) centre (0, 0) ccw
  line L0 (-5.596, 0.8992) -> (-5.3109, 0.6842)
  arc A2 (-5.3109, 0.6842) -> (-4.7295, 0.4406) centre (-4.5422, 1.7032) ccw
  arc A3 (-4.7295, 0.4406) -> (-4.7297, -0.4382) centre (0, 0) ccw
  arc A4 (-4.7297, -0.4382) -> (-5.5034, -0.8578) centre (-4.5671, -1.6611) ccw
  line L1 (-5.5034, -0.8578) -> (-5.5867, -0.955)
  arc A5 (-5.5867, -0.955) -> (-5.2959, -2.0192) centre (0, 0) ccw
  line L2 (-5.2959, -2.0192) -> (-4.9414, -2.0629)
  arc A6 (-4.9414, -2.0629) -> (-4.3162, -1.9832) centre (-4.7853, -0.7961) ccw
  arc A7 (-4.3162, -1.9832) -> (-3.877, -2.7443) centre (0, 0) ccw
  arc A8 (-3.877, -2.7443) -> (-4.3372, -3.4946) centre (-3.1247, -3.722) ccw
  line L3 (-4.3372, -3.4946) -> (-4.3608, -3.6204)
  arc A9 (-4.3608, -3.6204) -> (-3.5768, -4.3966) centre (0, 0) ccw
  line L4 (-3.5768, -4.3966) -> (-3.2479, -4.2572)
  arc A10 (-3.2479, -4.2572) -> (-2.7463, -3.8756) centre (-3.7461, -3.082) ccw
  arc A11 (-2.7463, -3.8756) -> (-1.9854, -4.3152) centre (0, 0) ccw
  arc A12 (-1.9854, -4.3152) -> (-2.0088, -5.195) centre (-0.845, -4.7857) ccw
  line L5 (-2.0088, -5.195) -> (-1.9663, -5.3157)
  arc A13 (-1.9663, -5.3157) -> (-0.8992, -5.596) centre (0, 0) ccw
  line L6 (-0.8992, -5.596) -> (-0.6842, -5.3109)
  arc A14 (-0.6842, -5.3109) -> (-0.4406, -4.7295) centre (-1.7032, -4.5422) ccw
  arc A15 (-0.4406, -4.7295) -> (0.4382, -4.7297) centre (0, 0) ccw
  arc A16 (0.4382, -4.7297) -> (0.8578, -5.5034) centre (1.6611, -4.5671) ccw
  line L7 (0.8578, -5.5034) -> (0.955, -5.5867)
  arc A17 (0.955, -5.5867) -> (2.0192, -5.2959) centre (0, 0) ccw
  line L8 (2.0192, -5.2959) -> (2.0629, -4.9414)
  arc A18 (2.0629, -4.9414) -> (1.9832, -4.3162) centre (0.7961, -4.7853) ccw
  arc A19 (1.9832, -4.3162) -> (2.7443, -3.877) centre (0, 0) ccw
  arc A20 (2.7443, -3.877) -> (3.4946, -4.3372) centre (3.722, -3.1247) ccw
  line L9 (3.4946, -4.3372) -> (3.6204, -4.3608)
  arc A21 (3.6204, -4.3608) -> (4.3966, -3.5768) centre (0, 0) ccw
  line L10 (4.3966, -3.5768) -> (4.2572, -3.2479)
  arc A22 (4.2572, -3.2479) -> (3.8756, -2.7463) centre (3.082, -3.7461) ccw
  arc A23 (3.8756, -2.7463) -> (4.3152, -1.9854) centre (0, 0) ccw
  arc A24 (4.3152, -1.9854) -> (5.195, -2.0088) centre (4.7857, -0.845) ccw
  line L11 (5.195, -2.0088) -> (5.3157, -1.9663)
  arc A25 (5.3157, -1.9663) -> (5.596, -0.8992) centre (0, 0) ccw
  line L12 (5.596, -0.8992) -> (5.3109, -0.6842)
  arc A26 (5.3109, -0.6842) -> (4.7295, -0.4406) centre (4.5422, -1.7032) ccw
  arc A27 (4.7295, -0.4406) -> (4.7297, 0.4382) centre (0, 0) ccw
  arc A28 (4.7297, 0.4382) -> (5.5034, 0.8578) centre (4.5671, 1.6611) ccw
  line L13 (5.5034, 0.8578) -> (5.5867, 0.955)
  arc A29 (5.5867, 0.955) -> (5.2959, 2.0192) centre (0, 0) ccw
  line L14 (5.2959, 2.0192) -> (4.9414, 2.0629)
  arc A30 (4.9414, 2.0629) -> (4.3162, 1.9832) centre (4.7853, 0.7961) ccw
  arc A31 (4.3162, 1.9832) -> (3.877, 2.7443) centre (0, 0) ccw
  arc A32 (3.877, 2.7443) -> (4.3372, 3.4946) centre (3.1247, 3.722) ccw
  line L15 (4.3372, 3.4946) -> (4.3608, 3.6204)
  arc A33 (4.3608, 3.6204) -> (3.5768, 4.3966) centre (0, 0) ccw
  line L16 (3.5768, 4.3966) -> (3.2479, 4.2572)
  arc A34 (3.2479, 4.2572) -> (2.7463, 3.8756) centre (3.7461, 3.082) ccw
  arc A35 (2.7463, 3.8756) -> (1.9854, 4.3152) centre (0, 0) ccw
  arc A36 (1.9854, 4.3152) -> (2.0088, 5.195) centre (0.845, 4.7857) ccw
  line L17 (2.0088, 5.195) -> (1.9663, 5.3157)
  arc A37 (1.9663, 5.3157) -> (0.8992, 5.596) centre (0, 0) ccw
  line L18 (0.8992, 5.596) -> (0.6842, 5.3109)
  arc A38 (0.6842, 5.3109) -> (0.4406, 4.7295) centre (1.7032, 4.5422) ccw
  arc A39 (0.4406, 4.7295) -> (-0.4382, 4.7297) centre (0, 0) ccw
  arc A40 (-0.4382, 4.7297) -> (-0.8578, 5.5034) centre (-1.6611, 4.5671) ccw
  line L19 (-0.8578, 5.5034) -> (-0.955, 5.5867)
  arc A41 (-0.955, 5.5867) -> (-2.0192, 5.2959) centre (0, 0) ccw
  line L20 (-2.0192, 5.2959) -> (-2.0629, 4.9414)
  arc A42 (-2.0629, 4.9414) -> (-1.9832, 4.3162) centre (-0.7961, 4.7853) ccw
  arc A43 (-1.9832, 4.3162) -> (-2.7443, 3.877) centre (0, 0) ccw
  arc A44 (-2.7443, 3.877) -> (-3.4946, 4.3372) centre (-3.722, 3.1247) ccw
  line L21 (-3.4946, 4.3372) -> (-3.6204, 4.3608)
  arc A45 (-3.6204, 4.3608) -> (-4.3966, 3.5768) centre (0, 0) ccw
  line L22 (-4.3966, 3.5768) -> (-4.2572, 3.2479)
  arc A46 (-4.2572, 3.2479) -> (-3.8756, 2.7463) centre (-3.082, 3.7461) ccw
  arc A47 (-3.8756, 2.7463) -> (-4.3152, 1.9854) centre (0, 0) ccw
  arc A48 (-4.3152, 1.9854) -> (-5.195, 2.0088) centre (-4.7857, 0.845) ccw
  line L23 (-5.195, 2.0088) -> (-5.3157, 1.9663)
  circle A49 centre (0, 0) radius 3.75
  circle A50 centre (0, 0) radius 1.5
  dimension "d76" = 7.5
  dimension "d77" = 3
  constraint concentric A0 A49
  constraint concentric A49 A50
  measures "d76" diameter of A49
  measures "d77" diameter of A50
extrude "Extrude12" cut sketch "Sketch11" against normal blind 1 contours A49 bodies 12